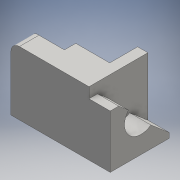
# Autodesk Inventor part: 240516_3Dsketch01
Saved by Autodesk Inventor 2016 (Build 200138000, 138)
## iProperties
Created: 2024-05-16
Part Number: 240516_3Dsketch01
Material: 일반
Document SubType Name: Modeling
Designer: pc
Density: 1 g/cm^3
Appearance: 기본값
Author: pc
Autodesk Inventor part; units mm, degrees
ref_plane "YZ Plane" through (0, 0, 0) normal (1, 0, 0) x (0, 1, 0)
ref_plane "XZ Plane" through (0, 0, 0) normal (0, 1, 0) x (-1, 0, 0)
ref_plane "XY Plane" through (0, 0, 0) normal (0, 0, 1) x (1, 0, 0)
sketch "스케치1" plane through (0, 0, 0) normal (0, 0, 1) x (1, 0, 0)
  line L0 (18.416, -13.8824) -> (-18.416, -13.8824)
  line L1 (-18.416, -13.8824) -> (-18.416, 13.8824)
  line L2 (-18.416, 13.8824) -> (18.416, 13.8824)
  line L3 (18.416, 13.8824) -> (18.416, -13.8824)
  line L4 (18.416, -13.8824) -> (-18.416, 13.8824) construction
  line L5 (-18.416, -13.8824) -> (18.416, 13.8824) construction
  point P0 (0, 0)
  constraints: 12 end point, 2 midpoint, 2 parallel, 1 horizontal, 1 perpendicular
extrude "돌출1" add sketch "스케치1" along normal blind 30
sketch "스케치2" plane through (18.416, -13.8824, 0) normal (1, 0, 0) x (0, 0, -1)
  line L0 (0, 27.7648) -> (0, 0) projected
  line L1 (0, 0) -> (-30, 0) projected
  line L2 (-25.0736, 0) -> (-25.0736, 4.0058)
  line L3 (-25.0736, 4.0058) -> (-21.1597, 8.5925)
  arc A0 (-21.1597, 8.5925) -> (-9.7848, 19.1723) centre (-16.0979, 14.5551) ccw
  line L4 (-9.7848, 19.1723) -> (-2.4526, 27.7648)
  line L5 (0, 27.7648) -> (-30, 27.7648) projected
  line L6 (0, 27.7648) -> (0, 0)
  point P0 (0, 13.8824)
  constraints: 8 end point, 2 perpendicular, 2 point on circle, 2 point on line, 1 centre point
extrude "돌출2" add sketch "스케치2" along normal blind 10
sketch "스케치3" plane through (-18.416, -13.8824, 0) normal (-1, 0, 0) x (0, 0, 1)
  line L0 (9.7848, 19.1723) -> (2.4526, 27.7648) projected
  line L1 (0, 27.7648) -> (30, 27.7648) projected
  line L2 (2.4526, 27.7648) -> (0, 27.7648)
  line L3 (0, 27.7648) -> (0, 6.044)
  line L4 (0, 0) -> (0, 27.7648) projected
  line L5 (30, 9.2244) -> (2.4526, 27.7648)
  line L6 (30, 9.2244) -> (30, 27.7648)
  point P0 (0, 13.8824)
  constraints: 8 end point, 1 collinear, 1 point on line, 1 vertical
extrude "돌출3" cut sketch "스케치3" against normal blind 16
sketch "스케치4" plane through (-2.416, -13.8824, 0) normal (-1, 0, 0) x (0, 0, 1)
  line L0 (2.4526, 27.7648) -> (30, 27.7648) projected
  line L1 (2.4526, 27.7648) -> (30, 14.5898)
  line L2 (30, 27.7648) -> (30, 9.2244) projected
  line L3 (30, 27.7648) -> (2.4526, 27.7648)
  point P0 (0, 13.8824)
  constraints: 4 end point, 1 perpendicular, 1 point on line
extrude "돌출4" cut sketch "스케치4" against normal blind 16
sketch "스케치5" plane through (-2.416, 0.7074, 30) normal (0, 0.9021329, 0.4314583) x (1, 0, 0)
  line L0 (0, -2.315) -> (0, 30.5359) projected
  line L1 (5.6646, 30.341) -> (0, 30.341)
  line L2 (0, 30.341) -> (0, 19.6839)
  line L3 (0, 19.6839) -> (5.6646, 19.6839)
  line L4 (5.6646, 19.6839) -> (5.6646, 30.341)
  point P0 (2.416, 26.7588)
  constraints: 8 end point, 2 parallel, 1 horizontal, 1 perpendicular, 1 point on line
extrude "돌출5" add sketch "스케치5" along normal blind 5
sketch "스케치6" plane through (-2.416, -13.8824, 0) normal (-1, 0, 0) x (0, 0, 1)
  line L0 (30, 14.5898) -> (2.4526, 27.7648) projected
  line L1 (12.2425, 23.0826) -> (14.3998, 27.5933) projected
  line L2 (2.6284, 27.6807) -> (14.3998, 27.5933)
  line L3 (4.7857, 32.1914) -> (14.3998, 27.5933) projected
  line L4 (14.3998, 27.5933) -> (4.7857, 32.1914)
  line L5 (4.7857, 32.1914) -> (2.6284, 27.6807)
  point P0 (0, 13.8824)
  constraints: 6 end point, 1 collinear, 1 perpendicular, 1 point on line
extrude "돌출6" cut sketch "스케치6" against normal blind 9 contours L5 L3 L2
sketch "스케치7" plane through (-2.416, -13.8824, 0) normal (-1, 0, 0) x (0, 0, 1)
  line L0 (12.2425, 23.0826) -> (14.3998, 27.5933) projected
  line L1 (14.3998, 27.5933) -> (12.2425, 23.0826)
  line L2 (12.2425, 23.0826) -> (12.2425, 27.6093)
  line L3 (14.3998, 27.5933) -> (2.6284, 27.6807) projected
  point P0 (0, 13.8824)
  constraints: 4 end point, 1 collinear, 1 point on line, 1 vertical
extrude "돌출7" cut sketch "스케치7" against normal blind 9
fillet "모깎기1" radius 4 1 edges at (-18.416, -9.2702, 30)
